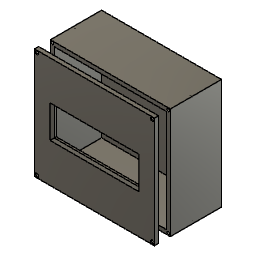
FireAlarmRx v2 (Autodesk Fusion 360 design; units mm, degrees)
part number: Configuración 1
Autodesk Fusion 360 part; units mm, degrees
note: some values were not read from the file. Set by a fixed rule: which sketch regions a step uses.
sketch "Boceto15" plane through (0, 0, 0) normal (0, 0, 1) x (1, 0, 0)
  line L0 (0, 0) -> (102, 0)
  line L1 (102, 0) -> (102, 94)
  line L2 (102, 94) -> (0, 94)
  line L3 (0, 94) -> (0, 0)
  line L4 (3.5, 90.4997) -> (98.5, 90.4997)
  line L5 (98.5, 90.4997) -> (98.5, 3.4997)
  line L6 (98.5, 3.4997) -> (3.5, 3.4997)
  line L7 (3.5, 3.4997) -> (3.5, 90.4997)
  dimension "d44" = 102
  dimension "d45" = 94
  dimension "d109" = 95
  dimension "d110" = 87
  constraint horizontal L0
  constraint vertical L1
  constraint horizontal L2
  constraint vertical L3
  constraint coincident L0.start L3.end
  constraint horizontal L4
  constraint vertical L5
  constraint horizontal L6
  constraint vertical L7
  measures "d44" distance of L0.start L0.end
  measures "d45" distance of L0.start L2.end
  measures "d109" distance of L4.start L4.end
  measures "d110" distance of L4.start L6.end
extrude "Extruir11" add sketch "Boceto15" against normal blind 3.5 contours L0 L1 L2 L3 | L4 L5 L6 L7 makes body 1
sketch "Boceto22" plane through (0, 0, 0) normal (0, 0, 1) x (1, 0, 0)
  circle A0 centre (1.7501, 1.7501) radius 1.1
  line L0 (0, 0) -> (102, 0)
  line L1 (102, 0) -> (102, 94)
  line L2 (102, 94) -> (0, 94)
  line L3 (0, 94) -> (0, 0)
  circle A1 centre (100.2499, 1.7501) radius 1.1
  circle A2 centre (100.2499, 92.2499) radius 1.1
  circle A3 centre (1.7501, 92.2499) radius 1.1
  line L4 (14.9998, 59) -> (86.9998, 59)
  line L5 (86.9998, 59) -> (86.9998, 35)
  line L6 (86.9998, 35) -> (14.9998, 35)
  line L7 (14.9998, 35) -> (14.9998, 59)
  dimension "d130" = 2.475
  dimension "d132" = 2.2
  dimension "d133" = 102
  dimension "d134" = 94
  dimension "d136" = 2.475
  dimension "d137" = 2.2
  dimension "d139" = 2.475
  dimension "d140" = 2.2
  dimension "d142" = 2.475
  dimension "d143" = 2.2
  dimension "d148" = 72
  dimension "d149" = 24
  constraint horizontal L0
  constraint vertical L1
  constraint horizontal L2
  constraint vertical L3
  constraint coincident L0.start L3.end
  constraint horizontal L4
  constraint vertical L5
  constraint horizontal L6
  constraint vertical L7
  measures "d130" distance of L0.start A0.centre
  measures "d132" diameter of A0
  measures "d133" distance of L0.start L0.end
  measures "d134" distance of L0.start L2.end
  measures "d136" distance of L0.end A1.centre
  measures "d137" diameter of A1
  measures "d139" distance of L1.end A2.centre
  measures "d140" diameter of A2
  measures "d142" distance of L2.end A3.centre
  measures "d143" diameter of A3
  measures "d148" distance of L4.start L4.end
  measures "d149" distance of L4.start L6.end
extrude "Extruir12" add sketch "Boceto15" along normal blind 40 bodies 1
move_body "Desplazar12" bodies 1 to x (1, 0, 0) y (0, 1, 0) z (0, 0, 1) at (0, 0, -40)
extrude "Extruir13" cut sketch "Boceto22" against normal blind 19 contours A0 | A1 | A2 | A3 bodies 1
extrude "Extruir14" add sketch "Boceto22" along normal blind 3.5 separate body makes body 2
move_body "Desplazar13" bodies 2 to x (1, 0, 0) y (0, 1, 0) z (0, 0, 1) at (0, 0, 10)
chamfer "Chaflán1" distance 1.8 angle 45 4 edges at (50.9998, 59, 13.5) (14.9998, 47, 13.5) (50.9998, 35, 13.5) (86.9998, 47, 13.5) on bodies 2
chamfer "Chaflán2" distance 0.5 angle 45 1 edges at (0.7245, 92.6477, 13.5) on bodies 2
chamfer "Chaflán3" distance 0.5 angle 45 1 edges at (99.2244, 92.6477, 13.5) on bodies 2
chamfer "Chaflán4" distance 0.5 angle 45 1 edges at (99.2244, 2.1479, 13.5) on bodies 2
chamfer "Chaflán5" distance 0.5 angle 45 1 edges at (0.7245, 2.1479, 13.5) on bodies 2
equation "d44 = 95 mm + ( 3.5 * 2 ) * 1 mm"
equation "d45 = 87 mm + ( 3.5 * 2 ) * 1 mm"
equation "d133 = 95 mm + ( 3.5 * 2 ) * 1 mm"
equation "d134 = 87 mm + ( 3.5 * 2 ) * 1 mm"
named bodies: "Box", "Cover"
